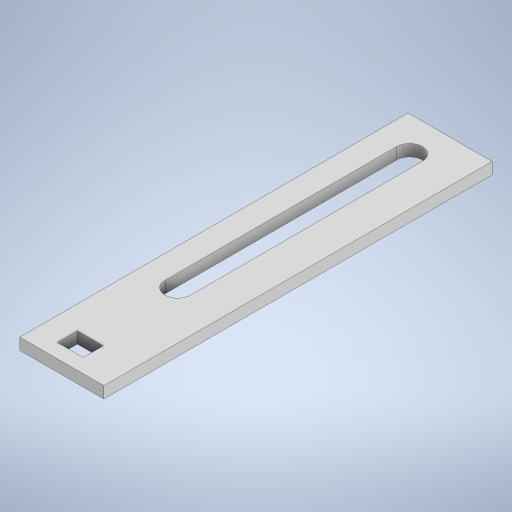
# Autodesk Inventor part: hammock_arms
Saved by Autodesk Inventor 2024.3 (Build 283343000, 343)
## iProperties
Created: 2024-08-04
Part Number: hammock_arms
Material: Generic
Document SubType Name: Modeling
Designer: compu
Density: 1 g/cm^3
Appearance: Default
Author: compu
Autodesk Inventor part; units mm, degrees
ref_plane "YZ Plane" through (0, 0, 0) normal (1, 0, 0) x (0, 1, 0)
ref_plane "XZ Plane" through (0, 0, 0) normal (0, 1, 0) x (-1, 0, 0)
ref_plane "XY Plane" through (0, 0, 0) normal (0, 0, 1) x (1, 0, 0)
sketch "Sketch2" plane through (0, 0, 0) normal (0, 1, 0) x (-1, 0, 0)
  line L0 (2.25, -1.75) -> (-2.25, -1.75)
  line L1 (-2.25, -1.75) -> (-2.25, 1.75)
  line L2 (-2.25, 1.75) -> (2.25, 1.75)
  line L3 (2.25, 1.75) -> (2.25, -1.75)
  line L4 (19.9632, 0) -> (-24.4134, 0) projected
  line L5 (0, -77.0314) -> (0, 22.3686) projected
  line L6 (6.25, 4.1686) -> (-8.25, 4.1686)
  line L7 (6.25, 4.1686) -> (6.25, -62.8314)
  line L8 (-8.25, 4.1686) -> (-8.25, -62.8314)
  line L9 (13.6237, 8.1686) -> (-18.0739, 8.1686) construction
  circle A0 centre (0, -36.8314) radius 2.2
  arc A1 (-2.2, -56.8314) -> (2.2, -56.8314) centre (0, -56.8314) ccw
  arc A2 (2.2, -16.8314) -> (-2.2, -16.8314) centre (0, -16.8314) ccw
  line L10 (2.2, -56.8314) -> (2.2, -16.8314)
  line L11 (-2.2, -56.8314) -> (-2.2, -16.8314)
  line L12 (6.25, -62.8314) -> (-8.25, -62.8314)
  point P0 (0, 0)
  dimension "d0" = 3.5
  dimension "d1" = 4.5
  dimension "d2" = 2.4186
  dimension "d3" = 4
  dimension "d4" = 6
  dimension "d5" = 4
  dimension "d6" = 4.4
  dimension "d7" = 45
  dimension "d8" = 4.4
  dimension "d9" = 4.4
  dimension "d10" = 20
  dimension "d11" = 20
  dimension "d12" = 6
  constraints: 22 end point, 4 horizontal, 4 point on circle, 4 vertical, 3 centre point, 3 point on line, 2 parallel, 2 tangent, 1 perpendicular, 2 other
  measures "d0" distance of L0.end L1.end
  measures "d1" distance of L0.start L0.end
  measures "d2" distance between parallel lines of L2 L6
  measures "d3" distance between parallel lines of L7 L3
  measures "d4" distance between parallel lines of L8 L1
  measures "d5" distance between parallel lines of L9 L6
  measures "d6" diameter of A0
  measures "d7" distance from line of L9 A0.centre
  measures "d8" diameter of A1
  measures "d9" diameter of A2
  measures "d10" distance of A0.centre A1.centre
  measures "d11" distance of A0.centre A2.centre
  measures "d12" distance from line of A1.centre L12
extrude "Extrusion1" add sketch "Sketch2" along normal blind 2 contours L3 L4 L7 L12 L5 A1 L10 A2 L0 | L5 A2 L11 A1 L12 L8 L4 L1 L0 | L3 L2 L5 L6 L7 L4 | L4 L8 L6 L5 L2 L1
body "Solid1"
